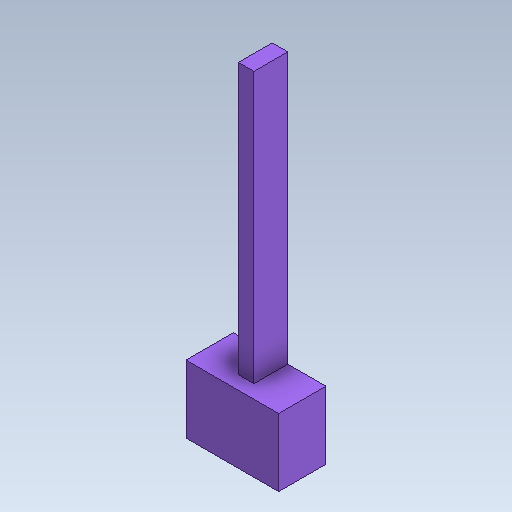
# Autodesk Inventor part: Piston
Saved by Autodesk Inventor 2020 (Build 240168000, 168)
## iProperties
Created: 2020-09-13
Part Number: Piston
Material: Generic
Document SubType Name: Modeling
Designer: Turing
Density: 1 g/cm^3
Appearance: Violet
Mass: 0.12705 g
Surface Area: 2.0595 cm^2
Volume: 0.12705 cm^3
Author: Turing
Autodesk Inventor part; units mm, degrees
ref_plane "YZ Plane" through (0, 0, 0) normal (1, 0, 0) x (0, 1, 0)
ref_plane "XZ Plane" through (0, 0, 0) normal (0, 1, 0) x (-1, 0, 0)
ref_plane "XY Plane" through (0, 0, 0) normal (0, 0, 1) x (1, 0, 0)
sketch "Sketch1" plane through (0, 0, 0) normal (0, 0, 1) x (1, 0, 0)
  line L0 (0, 0) -> (-3.45, 0)
  line L1 (-3.45, 0) -> (-3.45, -20)
  line L2 (-3.45, -20) -> (0, -20)
  line L3 (0, -20) -> (0, 0)
  line L4 (-1.725, -20) -> (-5.425, -20)
  line L5 (-5.425, -20) -> (1.925, -20)
  line L6 (1.925, -20) -> (1.925, -25)
  line L7 (1.925, -25) -> (-5.425, -25)
  line L8 (-5.425, -25) -> (-5.425, -20)
  dimension "d0" = 20
  dimension "d1" = 3.45
  dimension "d2" = 3.7
  dimension "d3" = 7.35
  dimension "d4" = 5
  constraints: 18 end point, 4 parallel, 3 horizontal, 2 perpendicular, 1 midpoint
  measures "d0" distance of L0.end L1.end
  measures "d1" distance of L0.start L0.end
  measures "d2" distance of L4.start L4.end
  measures "d3" distance of L6.end L7.end
  measures "d4" distance of L5.end L6.end
extrude "Extrusion1" add sketch "Sketch1" along normal blind 3.5
sketch "Sketch4" plane through (0, 0, 0) normal (0, 0, -1) x (-1, 0, 0)
  line L0 (0, -20) -> (0, 0) projected
  line L1 (-1.925, -20) -> (0, -20) projected
  line L2 (-1.925, -25) -> (-1.925, -20) projected
  line L3 (5.425, -25) -> (-1.925, -25) projected
  line L4 (5.425, -20) -> (5.425, -25) projected
  line L5 (3.45, -20) -> (5.425, -20) projected
  line L6 (3.45, 0) -> (3.45, -20) projected
  line L7 (0, 0) -> (3.45, 0) projected
  line L8 (3.45, 0) -> (5.475, 0)
  line L9 (0, 0) -> (-2.025, 0)
  line L10 (5.475, 0) -> (-2.025, 0)
  line L11 (-2.025, 0) -> (-2.025, 4)
  line L12 (-2.025, 4) -> (5.475, 4)
  line L13 (5.475, 4) -> (5.475, 0)
  circle A0 centre (1.725, 4) radius 3.75
  circle A1 centre (1.725, 4) radius 1.55
  dimension "d22" = 2.025
  dimension "d23" = 2.025
  dimension "d24" = 7.5
  dimension "d25" = 4
  dimension "d26" = 3.1
  constraints: 12 end point, 3 horizontal, 2 parallel, 1 centre point, 1 coincident, 1 midpoint, 1 perpendicular, 3 other
  measures "d22" distance of L6.start L8.end
  measures "d23" distance of L0.end L9.end
  measures "d24" distance of L11.end L12.end
  measures "d25" distance of L10.end L11.end
  measures "d26" diameter of A1
extrude "Extrusion4" add sketch "Sketch4" against normal up to surface (3.5 mm away) contours L9 L11 A0 L13 L8 L7 | A0 L12 A1 | L12 A1 A0
sketch "Sketch5" plane through (0, 0, 0) normal (0, 0, -1) x (-1, 0, 0)
  circle A0 centre (1.725, 4) radius 1.55 projected
  line L0 (0, -20) -> (0, 0) projected
  line L1 (-1.925, -20) -> (0, -20) projected
  line L2 (-1.925, -25) -> (-1.925, -20) projected
  line L3 (5.425, -25) -> (-1.925, -25) projected
  line L4 (5.425, -20) -> (5.425, -25) projected
  line L5 (3.45, -20) -> (5.425, -20) projected
  line L6 (3.45, 0) -> (3.45, -20) projected
  line L7 (3.45, 0) -> (5.475, 0) projected
  line L8 (5.475, 0) -> (5.475, 4) projected
  arc A1 (5.475, 4) -> (-2.025, 4) centre (1.725, 4) ccw projected
  line L9 (-2.025, 4) -> (-2.025, 0) projected
  line L10 (-2.025, 0) -> (0, 0) projected
  line L11 (3.45, -10) -> (0, -10)
  line L12 (2.45, -10) -> (2.45, -20)
  line L13 (1, -10) -> (1, -20)
  line L14 (3.45, -20) -> (2.45, -20)
  line L15 (1, -20) -> (0, -20)
  dimension "d29" = 1
  dimension "d30" = 1
  constraints: 10 end point, 2 midpoint, 2 point on line, 2 vertical, 1 horizontal, 1 perpendicular
  measures "d29" distance between parallel lines of L12 L6
  measures "d30" distance between parallel lines of L0 L13
extrude "Extrusion5" cut sketch "Sketch5" against normal up to surface (3.5 mm away) contours L0 L11 L13 L15 | L0 L10 L9 A1 L8 L7 L6 L11 | L11 L6 L14 L12
sketch "Sketch6" plane through (0, 0, 3.5) normal (0, 0, 1) x (1, 0, 0)
  line L0 (1.925, -20) -> (-1, -20) projected
  line L1 (-1, -20) -> (-1, -10) projected
  line L2 (-1, -10) -> (-2.45, -10) projected
  line L3 (-2.45, -10) -> (-2.45, -20) projected
  line L4 (-2.45, -20) -> (-5.425, -20) projected
  line L5 (-5.425, -20) -> (-5.425, -25) projected
  line L6 (-5.425, -25) -> (1.925, -25) projected
  line L7 (1.925, -25) -> (1.925, -20) projected
  line L8 (-1, -20) -> (-2.45, -20)
  point P0 (0, 0)
  constraints: 2 end point, 1 horizontal
extrude "Extrusion6" cut sketch "Sketch6" against normal blind 1.75 contours L8 L3 L2 L1
sketch "Sketch7" plane through (-5.425, -20, 3.5) normal (0, 1, 0) x (1, 0, 0)
  line L0 (4.425, 3.5) -> (7.35, 3.5) projected
  line L1 (4.425, 3.5) -> (4.425, 1.75) projected
  line L2 (4.425, 1.75) -> (2.975, 1.75) projected
  line L3 (2.975, 3.5) -> (2.975, 1.75) projected
  line L4 (0, 3.5) -> (2.975, 3.5) projected
  line L5 (0, 3.5) -> (0, 0) projected
  line L6 (7.35, 0) -> (0, 0) projected
  line L7 (7.35, 3.5) -> (7.35, 0) projected
  line L8 (0.5, 0.5) -> (0.5, 3)
  line L9 (0.5, 3) -> (2.475, 3)
  line L10 (2.475, 3) -> (2.475, 1.25)
  line L11 (2.475, 1.25) -> (4.925, 1.25)
  line L12 (4.925, 1.25) -> (4.925, 3)
  line L13 (4.925, 3) -> (6.85, 3)
  line L14 (6.85, 3) -> (6.85, 0.5)
  line L15 (6.85, 0.5) -> (0.5, 0.5)
  line L16 (2.475, 3) -> (4.925, 3)
  line L17 (2.975, 3.5) -> (4.425, 3.5)
  point P0 (5.425, 3.5)
  dimension "d35" = 0.5
  constraints: 20 end point, 2 horizontal, 7 other
  measures "d35" distance between parallel lines of L5 L8
extrude "Extrusion7" cut sketch "Sketch7" along normal blind 10 and the other way blind 2 contours L0 L7 L6 L5 L4 L3 L16 L9 L8 L15 L14 L13 L1 | L1 L16 L3 L17
sketch "Sketch8" plane through (-5.425, -22, 3.5) normal (0, 1, 0) x (1, 0, 0)
  line L0 (0, 3.5) -> (7.35, 3.5) projected
  line L1 (0, 0) -> (0, 3.5) projected
  line L2 (7.35, 0) -> (0, 0) projected
  line L3 (7.35, 3.5) -> (7.35, 0) projected
  line L4 (6.85, 3) -> (0.5, 3) projected
  line L5 (6.85, 0.5) -> (6.85, 3) projected
  line L6 (0.5, 0.5) -> (6.85, 0.5) projected
  line L7 (0.5, 3) -> (0.5, 0.5) projected
  point P0 (5.425, 3.5)
extrude "Extrusion8" add sketch "Sketch8" along normal up to surface (2 mm away)
sketch "Sketch9" plane through (-5.425, -20, 0) normal (0, 1, 0) x (1, 0, 0)
  line L0 (0, 0) -> (7.35, 0) projected
  line L1 (0, -3.5) -> (0, 0) projected
  line L2 (7.35, -3.5) -> (0, -3.5) projected
  line L3 (7.35, 0) -> (7.35, -3.5) projected
  line L4 (4.425, -0.5) -> (2.975, -0.5) projected
  line L5 (4.425, -0.5) -> (4.425, -1.75) projected
  line L6 (4.425, -1.75) -> (2.975, -1.75) projected
  line L7 (2.975, -0.5) -> (2.975, -1.75) projected
  line L8 (4.425, -0.5) -> (4.425, 0)
  line L9 (2.975, -0.5) -> (2.975, 0)
  point P0 (5.425, 0)
  constraints: 4 end point, 2 perpendicular, 2 point on line
extrude "Extrusion9" add sketch "Sketch9" along normal blind 10 contours L0 L8 L4 L9
sketch "Sketch10" plane through (0, 0, 1.75) normal (0, 0, 1) x (1, 0, 0)
  line L0 (-1, -20) -> (-2.45, -20) projected
  line L1 (-1, -10) -> (-1, -20) projected
  line L2 (-2.45, -10) -> (-1, -10) projected
  line L3 (-2.45, -20) -> (-2.45, -10) projected
  point P0 (0, 0)
extrude "Extrusion10" add sketch "Sketch10" along normal up to surface (1.75 mm away)
sketch "Sketch11" plane through (-2.45, -10, 0) normal (0, 1, 0) x (1, 0, 0)
  line L0 (0, 0) -> (0, -3.5) projected
  line L1 (0, -3.5) -> (1.45, -3.5) projected
  line L2 (1.45, 0) -> (1.45, -3.5) projected
  line L3 (1.45, 0) -> (0, 0) projected
  point P0 (2.45, 0)
extrude "Extrusion11" add sketch "Sketch11" along normal blind 10
sketch "Sketch12" plane through (0, 0, 3.5) normal (0, 0, 1) x (1, 0, 0)
  line L0 (-5.425, -20) -> (-5.425, -25) projected
  line L1 (-5.425, -25) -> (1.925, -25) projected
  line L2 (1.925, -25) -> (1.925, -20) projected
  line L3 (1.925, -20) -> (-1, -20) projected
  line L4 (-1, -20) -> (-1, 0) projected
  line L5 (-2.45, 0) -> (-1, 0) projected
  line L6 (-2.45, -20) -> (-2.45, 0) projected
  line L7 (-2.45, -20) -> (-5.425, -20) projected
  line L8 (-1.75, -25) -> (-5.425, -25)
  line L9 (-5.425, -25) -> (-5.325, -25)
  line L10 (-5.325, -25) -> (-5.325, -20)
  line L11 (-1.75, -25) -> (1.925, -25)
  line L12 (1.925, -25) -> (1.825, -25)
  line L13 (1.825, -25) -> (1.825, -20)
  point P0 (0, 0)
  dimension "d48" = 0.1
  dimension "d49" = 0.1
  constraints: 12 end point, 4 point on line, 2 collinear, 2 perpendicular, 1 midpoint
  measures "d48" distance of L0.end L9.end
  measures "d49" distance of L1.end L12.end
extrude "Extrusion12" cut sketch "Sketch12" against normal up to surface (3.5 mm away) contours L7 L10 L1 L0 | L13 L3 L2 L1
sketch "Sketch17" plane through (0, 0, 3.5) normal (0, 0, 1) x (1, 0, 0)
  line L0 (1.825, -25) -> (1.825, -20) projected
  line L1 (1.825, -20) -> (-1, -20) projected
  line L2 (-1, -20) -> (-1, 0) projected
  line L3 (-2.45, 0) -> (-1, 0) projected
  line L4 (-2.45, -20) -> (-2.45, 0) projected
  line L5 (-2.45, -20) -> (-5.325, -20) projected
  line L6 (-5.325, -20) -> (-5.325, -25) projected
  line L7 (-5.325, -25) -> (1.825, -25) projected
  line L8 (-1, -20) -> (-2.45, -20)
  point P0 (0, 0)
  constraints: 2 end point, 1 horizontal
extrude "Extrusion17" cut sketch "Sketch17" against normal blind 1 contours L8 L4 L3 L2
sketch "Sketch18" plane through (0, 0, 3.5) normal (0, 0, 1) x (1, 0, 0)
  line L0 (1.825, -20) -> (-5.325, -20) projected
  line L1 (-5.325, -20) -> (-5.325, -25) projected
  line L2 (-5.325, -25) -> (1.825, -25) projected
  line L3 (1.825, -25) -> (1.825, -20) projected
  line L4 (1.825, -25) -> (1.675, -25)
  line L5 (1.675, -25) -> (1.675, -20)
  line L6 (-5.325, -25) -> (-5.175, -25)
  line L7 (-5.175, -25) -> (-5.175, -20)
  point P0 (0, 0)
  dimension "d65" = 0.15
  dimension "d66" = 0.15
  constraints: 8 end point, 4 point on line, 2 perpendicular
  measures "d65" distance of L2.end L4.end
  measures "d66" distance of L1.end L6.end
extrude "Extrusion18" cut sketch "Sketch18" against normal up to surface (3.5 mm away) contours L3 L2 L5 L0 | L7 L2 L1 L0
sketch "Sketch19" plane through (0, 0, 2.5) normal (0, 0, 1) x (1, 0, 0)
  line L0 (-2.45, 0) -> (-1, 0) projected
  line L1 (-2.45, -20) -> (-2.45, 0) projected
  line L2 (-1, -20) -> (-2.45, -20) projected
  line L3 (-1, 0) -> (-1, -20) projected
  line L4 (-1.725, 0) -> (-2.45, 0)
  line L5 (-2.45, 0) -> (-2.3, 0)
  line L6 (-2.3, 0) -> (-2.3, -20)
  line L7 (-1, -20) -> (-1.15, -20)
  line L8 (-1.15, -20) -> (-1.15, 0)
  point P0 (0, 0)
  dimension "d69" = 0.15
  dimension "d70" = 0.15
  constraints: 10 end point, 4 point on line, 2 perpendicular, 1 collinear, 1 midpoint
  measures "d69" distance of L0.start L5.end
  measures "d70" distance of L2.start L7.end
extrude "Extrusion19" cut sketch "Sketch19" against normal up to surface (2.5 mm away) contours L0 L6 L2 L1 | L0 L3 L2 L8
equation "\"d23\" = d22"
equation "\"d30\" = d29"
equation "\"d49\" = d48"
equation "\"d69\" = d70"
body "Solid1"
